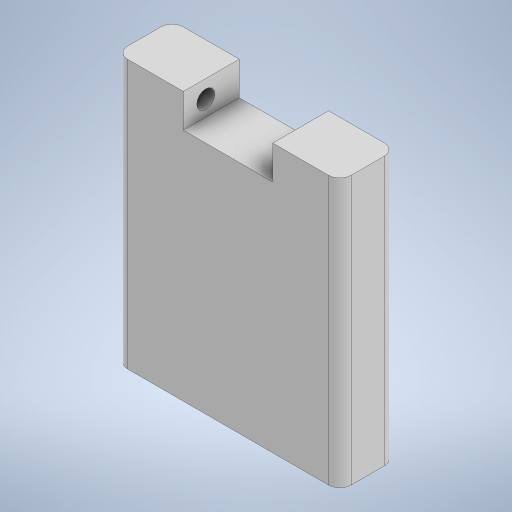
# Autodesk Inventor part: Bauteil5
Saved by Autodesk Inventor 2023 (Build 270158000, 158)
## iProperties
Created: 2024-02-03
Part Number: Bauteil5
Material: Generisch
Document SubType Name: Modeling
Designer: jefar
Density: 1 g/cm^3
Appearance: Vorgabe
Author: jefar
Autodesk Inventor part; units mm, degrees
ref_plane "YZ Plane" through (0, 0, 0) normal (1, 0, 0) x (0, 1, 0)
ref_plane "XZ Plane" through (0, 0, 0) normal (0, 1, 0) x (-1, 0, 0)
ref_plane "XY Plane" through (0, 0, 0) normal (0, 0, 1) x (1, 0, 0)
sketch "Skizze1" plane through (0, 0, 0) normal (0, 0, 1) x (1, 0, 0)
  line L0 (-7000, 0) -> (7000, 0) construction
  line L1 (0, -8400) -> (0, 8400) construction
  line L2 (-5000, -6000) -> (5000, -6000)
  line L3 (5000, -6000) -> (5000, 6000)
  line L4 (5000, 6000) -> (-5000, 6000)
  line L5 (-5000, 6000) -> (-5000, -6000)
  line L6 (-5000, -6000) -> (5000, 6000) construction
  line L7 (5000, -6000) -> (-5000, 6000) construction
  line L8 (5000, 6000) -> (2000, 6000)
  line L9 (5000, 4500) -> (5000, 6000)
  line L10 (-5000, 6000) -> (-5000, 6000)
  line L11 (-5000, 6000) -> (-5000, 4500)
  line L12 (5000, 6000) -> (2000, 6000)
  line L13 (2000, 6000) -> (2000, 4500)
  line L14 (5000, 4500) -> (5000, 6000)
  line L15 (-5000, 6000) -> (-2000, 6000)
  line L16 (-2000, 6000) -> (-2000, 4500)
  line L17 (-5000, 4500) -> (-5000, 6000)
  line L18 (-2000, 4500) -> (2000, 4500)
  point P0 (0, 0)
  dimension "d5" = 12000
  dimension "d6" = 3000
  dimension "d7" = 3000
  constraints: 34 end point, 6 horizontal, 4 parallel, 4 perpendicular, 2 midpoint
  measures "d5" distance of L2.end L3.end
  measures "d6" distance of L14.start L13.end
  measures "d7" distance of L16.end L17.start
extrude "Extrusion1" add sketch "Skizze1" along normal blind 2500 contours L5 L4 L16 L18 L13 L3 L2
sketch "Skizze2" plane through (-2000, 4500, 0) normal (1, 0, 0) x (0, 0, -1)
  circle A0 centre (-1500, 700) radius 400
  line L0 (0, -10500) -> (0, 1500) construction
  line L1 (0, 0) -> (-2500, 0) construction
  point P0 (0, -4500)
  point P1 (-1250, 0)
  constraints: 1 centre point, 1 midpoint
extrude "Extrusion2" cut sketch "Skizze2" against normal blind 2000
extrude "Extrusion3" cut sketch "Skizze2" along normal blind 6000
sketch "Skizze3" plane through (-5000, -6000, 0) normal (-1, 0, 0) x (0, 0, 1)
  point P0 (0, 6000)
fillet "Rundung1" radius 500 4 edges at (-5000, 0, 0) (-5000, 0, 2500) (5000, 0, 0) (5000, 0, 2500)
